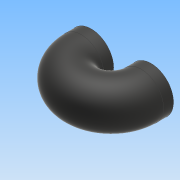
# Autodesk Inventor part: Pancake_Flexi Pipe
Saved by Autodesk Inventor 2018.1 (Build 221171000, 171)
## iProperties
Created: 2019-02-26
Part Number: Pancake_Flexi Pipe
Material: PVC-Piping
Document SubType Name: Modeling
Designer: James
Density: 1.4 g/cm^3
Appearance: Smooth - Black
Author: James
Autodesk Inventor part; units mm, degrees
ref_plane "YZ Plane" through (0, 0, 0) normal (1, 0, 0) x (0, 1, 0)
ref_plane "XZ Plane" through (0, 0, 0) normal (0, 1, 0) x (-1, 0, 0)
ref_plane "XY Plane" through (0, 0, 0) normal (0, 0, 1) x (1, 0, 0)
sketch "Sketch1" plane through (0, 0, 0) normal (0, 1, 0) x (-1, 0, 0)
  circle A0 centre (0, 0) radius 20
  circle A1 centre (0, 0) radius 22.5
  dimension "d0" = 40
  dimension "d1" = 45
  constraints: 2 centre point, 2 coincident
  measures "d0" diameter of A0
  measures "d1" diameter of A1
sketch "Sketch2" plane through (0, 0, 0) normal (0, 0, 1) x (1, 0, 0)
  arc A0 (-60, 0) -> (0, 0) centre (-30, 0) ccw
  dimension "d8" = 30
  constraints: 2 horizontal alignment, 2 point on circle, 1 centre point
  measures "d8" distance of A0.end A0.centre
sweep "Sweep2" add profiles "Sketch1" path "Sketch2"
sketch "Sketch3" plane through (-60, 0, 0) normal (0, 1, 0) x (1, 0, 0)
  circle A0 centre (0, 0) radius 20 projected
  circle A1 centre (0, 0) radius 22.5 projected
  circle A2 centre (60, 0) radius 20 projected
  circle A3 centre (60, 0) radius 22.5 projected
extrude "Extrusion1" add sketch "Sketch3" along normal blind 10
body "Solid2"
